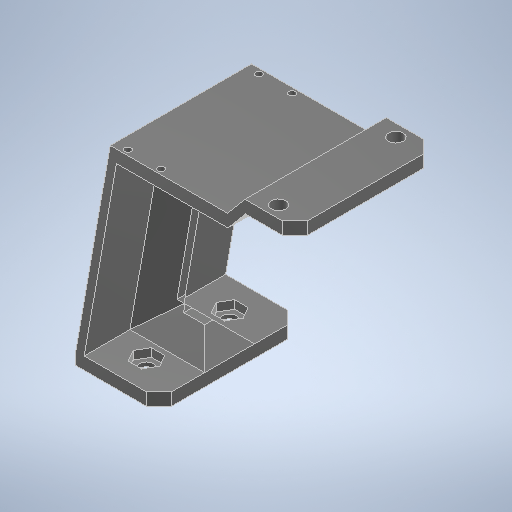
# Autodesk Inventor part: 3D_camera-fix-r2
Saved by Autodesk Inventor 2025 (Build 290162000, 162)
## iProperties
Created: 2024-06-30
Part Number: 3D_camera-fix-r2
Material: 一般
Document SubType Name: Modeling
Designer: 8326d
Density: 1 g/cm^3
Appearance: 滑らか - 黒
Author: 8326d
## iProperties of the stored document 3D_camera-fix-r2_3D プリント.ipt
Created: 2024-08-17
Part Number: 3D_camera-fix-r2_3D プリント
Material: 一般
Document SubType Name: Modeling
Designer: 8326d
Density: 1 g/cm^3
Appearance: 既定
Author: 8326d
Autodesk Inventor part; units mm, degrees
ref_plane "YZ Plane" through (0, 0, 0) normal (1, 0, 0) x (0, 1, 0)
ref_plane "XZ Plane" through (0, 0, 0) normal (0, 1, 0) x (-1, 0, 0)
ref_plane "XY Plane" through (0, 0, 0) normal (0, 0, 1) x (1, 0, 0)
sketch "スケッチ1" plane through (0, 0, 0) normal (0, 0, 1) x (1, 0, 0)
  line L0 (120.5, 0) -> (-120.5, 0) construction
  line L1 (120.5, 0) -> (361.5, 0) construction
  line L2 (-120.5, 0) -> (-100.5, 0)
  line L3 (-100.5, 0) -> (-100.5, 3)
  line L4 (-100.5, 3) -> (-120.5, 3)
  line L5 (-120.5, 3) -> (-120.5, 0)
  line L6 (-120.5, 3) -> (-60.5, 3) construction
  line L7 (-79.8, 54.961524) -> (-67.8, 54.961524)
  line L8 (-67.8, 54.961524) -> (-67.8, 51.961524)
  line L9 (-67.8, 51.961524) -> (-79.8, 51.961524)
  line L10 (-79.8, 51.961524) -> (-79.8, 54.961524)
  line L11 (-118.469147, 3) -> (-110.717544, 46.961524)
  line L12 (-110.717544, 46.961524) -> (-83.901982, 46.961524)
  line L13 (-83.901982, 46.961524) -> (-79.706484, 51.961524)
  line L14 (-79.8, 54.961524) -> (-83.995498, 49.961524)
  line L15 (-83.995498, 49.961524) -> (-112.219416, 49.961524)
  line L16 (-112.219416, 49.961524) -> (-120.5, 3)
  point P0 (0, 0)
  point P1 (0, 0)
  point P2 (-118.469147, 3)
  dimension "d0" = 241
  dimension "d1" = 180
  dimension "d2" = 20
  dimension "d3" = 3
  dimension "d6" = 12
  dimension "d7" = 3
  dimension "d72" = 2
  dimension "d74" = 3
  dimension "d75" = 40.7
  dimension "d89" = 5
  dimension "d92" = 51.96152
  dimension "d93" = 80
  dimension "d94" = 2
  dimension "d95" = 130
  constraints: 34 end point, 7 parallel, 6 horizontal, 2 perpendicular, 2 point on line, 1 coincident, 1 collinear, 1 midpoint
  measures "d0" distance of L0.start L0.end
  measures "d1" angle of L0 L1
  measures "d2" distance of L4.end L3.end
  measures "d3" distance of L3.end L2.end
  measures "d6" distance of L8.end L9.end
  measures "d7" distance of L7.end L8.end
  measures "d72" distance between parallel lines of L14 L13
  measures "d74" distance between parallel lines of L12 L15
  measures "d75" distance between parallel lines of L5 L10
  measures "d89" distance between parallel lines of L7 L15
  measures "d92" distance between parallel lines of L6 L7
  measures "d93" angle of L6 L16
  measures "d94" distance between parallel lines of L16 L11
  measures "d95" angle of L7 L14
extrude "押し出し1" add sketch "スケッチ1" along normal mid plane 34
sketch "スケッチ2" plane through (0, 0, 0) normal (0, 0, 1) x (1, 0, 0)
  line L0 (-100.5, 3) -> (-120.5, 3)
  line L1 (-100.5, 3) -> (-105.5, 8)
  line L2 (-105.5, 8) -> (-112.510379, 8)
  line L3 (-77.374946, 46.961524) -> (-72.8, 46.961524)
  line L4 (-72.8, 46.961524) -> (-67.8, 51.961524)
  line L5 (-79.706484, 51.961524) -> (-83.901982, 46.961524)
  line L6 (-83.901982, 46.961524) -> (-110.717544, 46.961524)
  line L7 (-110.717544, 46.961524) -> (-118.469147, 3)
  line L8 (-77.374946, 46.961524) -> (-81.570444, 41.961524)
  line L9 (-81.570444, 41.961524) -> (-106.522046, 41.961524)
  line L10 (-106.522046, 41.961524) -> (-112.510379, 8)
  line L11 (-67.8, 51.961524) -> (-79.706484, 51.961524)
  point P0 (0, 0)
  point P1 (-118.190599, 3)
  point P2 (-118.469147, 3)
  dimension "d13" = 5
  dimension "d14" = 45
  dimension "d76" = 5
  dimension "d77" = 45
  dimension "d78" = 5
  constraints: 14 end point, 1 horizontal, 1 parallel, 3 other
  measures "d13" distance between parallel lines of L0 L2
  measures "d14" angle of L0 L1
  measures "d76" distance between parallel lines of L11 L3
  measures "d77" angle of L11 L4
  measures "d78" distance between parallel lines of L5 L8
extrude "押し出し2" add sketch "スケッチ2" along normal mid plane 2
chamfer "面取り1" distance 5 angle 45 10 edges at (-109.4846, 3, 1) (-109.4846, 3, -1) (-73.7532, 51.9615, -1) (-73.7532, 51.9615, 1) (-81.8042, 49.4615, -1) (-97.3098, 46.9615, -1) (-114.5933, 24.9808, -1) (-81.8042, 49.4615, 1) (-97.3098, 46.9615, 1) (-114.5933, 24.9808, 1)
chamfer "面取り2" distance 2 angle 45 4 edges at (-112.5104, 8, 0) (-77.3749, 46.9615, 0) (-106.522, 41.9615, 0) (-81.5704, 41.9615, 0)
sketch "スケッチ3" plane through (-120.5, 0, 17) normal (0, -1, 0) x (1, 0, 0)
  line L0 (10, -7) -> (10, -27) construction
  line L1 (10, -7) -> (30, -7) construction
  line L2 (0, -34) -> (0, 0) construction
  point P0 (120.5, -17)
  point P1 (10, -17)
  point P2 (0, -17)
  dimension "d24" = 20
  dimension "d25" = 90
  dimension "d26" = 10
  constraints: 4 end point, 2 midpoint, 1 horizontal, 1 horizontal alignment, 1 perpendicular, 1 vertical
  measures "d24" distance of L0.start L0.end
  measures "d25" angle of L0 L1
  measures "d26" distance between parallel lines of L2 L0
hole "穴1" at (-110.5, 0, 10) at (-110.5, 0, -10) direction (0, 1, 0) diameter 3.5 depth 4 tip angle 118
sketch "スケッチ4" plane through (-100.5, 3, 17) normal (0, 1, 0) x (1, 0, 0)
  circle A0 centre (-10, 27) radius 1.75
  circle A1 centre (-10, 7) radius 1.75
  line L0 (-6.766838, 7) -> (-8.383419, 4.2)
  line L1 (-8.383419, 4.2) -> (-11.616581, 4.2)
  line L2 (-11.616581, 4.2) -> (-13.233162, 7)
  line L3 (-13.233162, 7) -> (-11.616581, 9.8)
  line L4 (-11.616581, 9.8) -> (-8.383419, 9.8)
  line L5 (-8.383419, 9.8) -> (-6.766838, 7)
  line L6 (-6.766838, 27) -> (-8.383419, 24.2)
  line L7 (-8.383419, 24.2) -> (-11.616581, 24.2)
  line L8 (-11.616581, 24.2) -> (-13.233162, 27)
  line L9 (-13.233162, 27) -> (-11.616581, 29.8)
  line L10 (-11.616581, 29.8) -> (-8.383419, 29.8)
  line L11 (-8.383419, 29.8) -> (-6.766838, 27)
  point P0 (100.5, 17)
  point P1 (-11.75, 30)
  point P2 (-8.25, 30)
  point P3 (-8.25, 0)
  point P4 (-11.75, 0)
  dimension "d34" = 5.6
  dimension "d35" = 5.6
  constraints: 24 end point, 2 coincident, 2 horizontal alignment, 28 other
  measures "d34" distance between parallel lines of L7 L10
  measures "d35" distance between parallel lines of L4 L1
extrude "押し出し3" cut sketch "スケッチ4" against normal blind 2 contours A0 | A1 | L0 L1 L2 L3 L4 L5 | L6 L7 L8 L9 L10 L11
sketch "スケッチ5" plane through (-79.8, 54.961524, 17) normal (0, 1, 0) x (1, 0, 0)
  line L0 (5.2, 31.1) -> (5.2, 2.9) construction
  line L1 (5.2, 31.1) -> (33.4, 31.1) construction
  line L2 (12, 34) -> (12, 0) construction
  line L3 (0, 34) -> (0, 0) projected
  point P0 (79.8, 17)
  point P1 (5.2, 17)
  dimension "d38" = 28.2
  dimension "d39" = 90
  dimension "d90" = 5.2
  constraints: 4 end point, 1 horizontal, 1 horizontal alignment, 1 midpoint, 1 perpendicular, 1 vertical
  measures "d38" distance of L0.start L0.end
  measures "d39" angle of L0 L1
  measures "d90" distance between parallel lines of L3 L0
hole "穴2" at (-74.6, 54.961524, -14.1) at (-74.6, 54.961524, 14.1) direction (0, -1, 0) diameter 3.5 depth 8 tip angle 118
chamfer "面取り4" distance 3 angle 45 4 edges at (-67.8, 53.4615, -17) (-67.8, 53.4615, 17) (-100.5, 1.5, -17) (-100.5, 1.5, 17)
sketch "スケッチ10" plane through (-112.219416, 49.961524, 17) normal (0, 1, 0) x (1, 0, 0)
  line L0 (11, 32.75) -> (3, 32.75) construction
  line L1 (3, 32.75) -> (3, 1.25) construction
  line L2 (3, 1.25) -> (11, 1.25) construction
  line L3 (11, 1.25) -> (11, 32.75) construction
  line L4 (11, 32.75) -> (3, 1.25) construction
  line L5 (3, 32.75) -> (11, 1.25) construction
  line L6 (44.419416, 31) -> (44.419416, 3) construction
  line L7 (28.223918, 34) -> (28.223918, 0) construction
  line L8 (0, 34) -> (0, 0)
  point P0 (112.219416, 17)
  point P1 (7, 17)
  point P2 (44.419416, 17)
  dimension "d79" = 8
  dimension "d80" = 31.5
  dimension "d96" = 3
  constraints: 12 end point, 3 midpoint, 2 parallel, 1 horizontal, 1 horizontal alignment, 1 perpendicular
  measures "d79" distance of L2.end L1.end
  measures "d80" distance of L1.end L0.end
  measures "d96" distance between parallel lines of L8 L1
hole "穴4" at (-109.219416, 49.961524, -15.75) at (-101.219416, 49.961524, -15.75) at (-101.219416, 49.961524, 15.75) at (-109.219416, 49.961524, 15.75) direction (0, -1, 0) diameter 1.6 depth 8 tip angle 118
equation "\"d7\" = d3"
equation "\"d72\" = d94"
equation "\"d13\" = d76"
equation "\"d77\" = d14"
equation "\"d35\" = d34"
